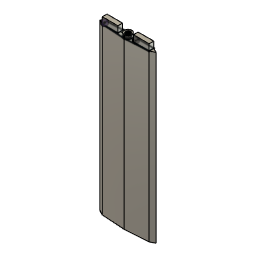
せんたーぼーど v1 (Autodesk Fusion 360 design; units mm, degrees)
Autodesk Fusion 360 part; units mm, degrees
note: some values were not read from the file. Set by a fixed rule: which face or edge a step refers to.
sketch "スケッチ1" plane through (0, 0, 0) normal (0, 1, 0) x (1, 0, 0)
  line L0 (0, 1.5) -> (10, 1.5)
  line L1 (10, 1.5) -> (10, -1.5)
  line L2 (10, -1.5) -> (0, -1.5)
  line L3 (0, -1.5) -> (0, 1.5)
  line L4 (20, 1.5) -> (30, 1.5)
  line L5 (30, 1.5) -> (30, -1.5)
  line L6 (30, -1.5) -> (20, -1.5)
  line L7 (20, -1.5) -> (20, 1.5)
  line L8 (10, 0) -> (20, 0) construction
  circle A0 centre (15, 0) radius 1.5
  circle A1 centre (15, 0) radius 2.5
  line L9 (0, -1.5) -> (15, -2.5)
  line L10 (15, -2.5) -> (30, -1.5)
  line L11 (30, 1.5) -> (15, 2.5)
  line L12 (15, 2.5) -> (0, 1.5)
  point P0 (20, 0)
  dimension "d1" = 10
  dimension "d2" = 3
  dimension "d3" = 10
  dimension "d4" = 3
  dimension "d5" = 10
  dimension "d6" = 3
  dimension "d8" = 5
  constraint horizontal L0
  constraint vertical L1
  constraint horizontal L2
  constraint vertical L3
  constraint horizontal L4
  constraint vertical L5
  constraint horizontal L6
  constraint vertical L7
  constraint midpoint L3 origin
  constraint midpoint L7 P0
  constraint horizontal origin P0
  constraint midpoint L1 L8.start
  constraint coincident P0 L8.end
  constraint midpoint L8 A0.centre
  constraint coincident A1 L9.end
  constraint vertical A0.centre L9.end
  constraint coincident A1 L11.end
  constraint vertical A0.centre L11.end
  measures "d1" distance of L0.start L0.end
  measures "d2" distance of L0.start L2.end
  measures "d3" distance of L4.start L4.end
  measures "d4" distance of L4.start L6.end
  measures "d5" distance of L1 L7
  measures "d6" diameter of A0
  measures "d8" diameter of A1
extrude "押し出し1" add sketch "スケッチ1" along normal blind 2 contours L0 L1 L2 L3 | A1 L9 L10 L11 L12 | L4 L5 L6 L7 makes body 1 at (3.3333, 0, -0.5) makes body 2 at (16.4981, 1.3333, 0.0748) makes body 3 at (23.3333, 0, -0.5)
extrude "押し出し2" add sketch "スケッチ1" against normal blind 6 contours L0 L1 L2 A1 L9 L12 | L0 L1 L2 L3 | A1 L9 L10 L11 L12 | L4 L6 L7 A1 L10 L11 | L4 L5 L6 L7 bodies 1 2 3
thread "ねじ1" "ISO Metric profile 3.0 M3x0.5 M3x0.5 6H" major diameter 3.086 minor diameter 2.529 pitch 0.5 angle 60 modelled right hand crest width 0.1368 on face at (16.4981, -4, 0.0748) crest through (16.2645, -5.875, 0) on face at (16.4981, 1.3333, 0.0748) crest through (16.2645, -5.875, 0) on bodies 1
extrude "押し出し3" add sketch "スケッチ1" against normal blind 100 from surface at -6 contours L0 L1 L2 A1 L9 L12 | L0 L1 L2 L3 | A1 L9 L10 L11 L12 | L4 L6 L7 A1 L10 L11 | L4 L5 L6 L7 | A0 bodies 1
sketch "スケッチ4" plane through (0, 0, 0) normal (0, 1, 0) x (1, 0, 0)
  line L0 (15, 2.5) -> (0, 1.5)
  line L1 (0, -1.5) -> (15, -2.5)
  line L2 (15, -2.5) -> (30, -1.5)
  line L3 (30, 1.5) -> (15, 2.5)
  line L4 (0, 1.5) -> (-3, 0)
  line L5 (-3, 0) -> (0, -1.5)
  line L6 (30, 1.5) -> (33, 0)
  line L7 (33, 0) -> (30, -1.5)
  line L8 (30, 1.5) -> (30, -1.5)
  line L9 (0, 1.5) -> (0, -1.5)
  dimension "d19" = 3
  dimension "d20" = 3
  constraint coincident L0.end L4.start
  constraint coincident L1.start L5.end
  constraint coincident L3.start L6.start
  constraint parallel L5 L6
  constraint coincident L2.end L7.end
  constraint parallel L4 L7
  measures "d19" distance of L4.end origin
  measures "d20" distance of L6.end L8
extrude "押し出し4" add sketch "スケッチ4" against normal up to surface (106 mm away) contours L4 L5 L9 | L6 L7 L8 bodies 1
extrude "押し出し5" add 2 faces at (3.3333, 2, -0.5) (23.3333, 2, -0.5) along direction (0, 1, 0) blind 2 on bodies 1 bodies 1
equation "d20 = d19"
